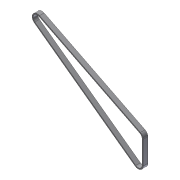
# Autodesk Inventor part: ShooterBelt
Saved by Autodesk Inventor 2012 (Build 160160000, 160)
## iProperties
Created: 2012-02-23
Part Number: ShooterBelt
Material: Rubber
Document SubType Name: Modeling
Designer: JesseK
Mass: 24.0647 g
Surface Area: 213.934 cm^2
Volume: 25.8761 cm^3
Density: 0.93 g/cm^3
Author: JesseK
Autodesk Inventor part; units mm, degrees
ref_plane "YZ Plane" through (0, 0, 0) normal (1, 0, 0) x (0, 1, 0)
ref_plane "XZ Plane" through (0, 0, 0) normal (0, 1, 0) x (-1, 0, 0)
ref_plane "XY Plane" through (0, 0, 0) normal (0, 0, 1) x (1, 0, 0)
sketch "Sketch1" plane through (0, 0, 0) normal (0, 0, 1) x (1, 0, 0)
  arc A0 (1.8788, 9.9306) -> (-9.665, -8.9721) centre (-3.1084, 0) ccw
  arc A1 (287.3193, -140.2716) -> (281.1939, -130.341) centre (276.2068, -140.2716) ccw
  arc A2 (269.6501, -213.0916) -> (287.3193, -204.1195) centre (276.2068, -204.1195) ccw
  line L0 (1.8788, 9.9306) -> (281.1939, -130.341)
  line L1 (287.3193, -140.2716) -> (287.3193, -204.1195)
  line L2 (269.6501, -213.0916) -> (-9.665, -8.9721)
  arc A3 (3.3036, 12.7679) -> (-11.5383, -11.5355) centre (-3.1084, 0) ccw
  arc A4 (290.4943, -140.2716) -> (282.6188, -127.5037) centre (276.2068, -140.2716) ccw
  arc A5 (267.7768, -215.655) -> (290.4943, -204.1195) centre (276.2068, -204.1195) ccw
  line L3 (290.4943, -140.2716) -> (290.4943, -204.1195)
  line L4 (-11.5383, -11.5355) -> (267.7768, -215.655)
  line L5 (282.6188, -127.5037) -> (3.3036, 12.7679)
  point P0 (0, 0)
  dimension "d0" = 11.1125
  dimension "d1" = 3.175
  constraints: 12 end point, 12 point on circle, 12 tangent, 6 centre point, 3 coincident, 2 equal radius, 2 parallel
  measures "d0" radius of A1
  measures "d1" distance between parallel lines of L2 L4
extrude "Extrusion1" add sketch "Sketch1" along normal blind 10.16
body "Solid1"
